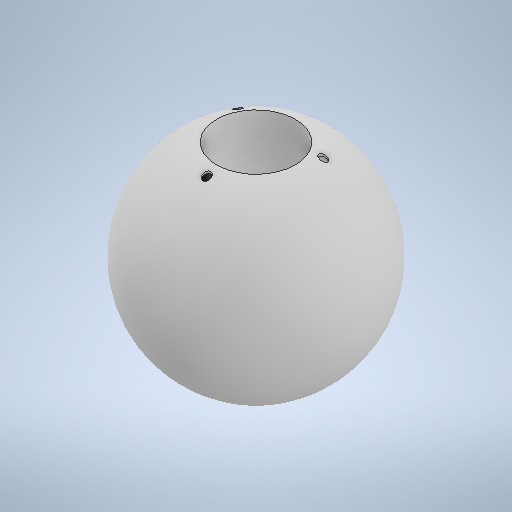
# Autodesk Inventor part: Buoy 10 2in Sphere
Saved by Autodesk Inventor 2025 (Build 290162000, 162)
## iProperties
Created: 2024-07-08
Part Number: Buoy 10 2in Sphere
Material: Generic
Document SubType Name: Modeling
Designer: track
Density: 1 g/cm^3
Appearance: Default
Mass: 1796.3 g
Surface Area: 1146.89 cm^2
Volume: 1796.3 cm^3
Author: track
## iProperties of the stored document Buoy 10 2in Sphere_3DPrint.ipt
Created: 2024-07-08
Part Number: Buoy 10 2in Sphere_3DPrint
Material: Generic
Document SubType Name: Modeling
Designer: track
Density: 1 g/cm^3
Appearance: Default
Author: track
Autodesk Inventor part; units mm, degrees
ref_plane "YZ Plane" through (0, 0, 0) normal (1, 0, 0) x (0, 1, 0)
ref_plane "XZ Plane" through (0, 0, 0) normal (0, 1, 0) x (-1, 0, 0)
ref_plane "XY Plane" through (0, 0, 0) normal (0, 0, 1) x (1, 0, 0)
sketch "Sketch1" plane through (0, 0, 0) normal (0, 0, 1) x (1, 0, 0)
  line L0 (0, 0) -> (0, 152.4)
  line L1 (0, 152.4) -> (30.48, 152.4) construction
  line L2 (30.48, 152.4) -> (30.48, 0)
  arc A0 (30.48, 0) -> (30.48, 152.4) centre (-1.27, 76.2) ccw
  line L3 (31.98, 2.2842) -> (31.98, 150.1158)
  arc A1 (31.98, 2.2842) -> (31.98, 150.1158) centre (-1.27, 76.2) ccw
  point P0 (81.28, 76.2)
  dimension "d0" = 152.4
  dimension "d1" = 30.48
  dimension "d2" = 50.8
  dimension "d3" = 0
  dimension "d4" = 1.5
  constraints: 8 end point, 5 point on circle, 2 centre point, 2 perpendicular, 1 vertical, 1 other
  measures "d0" distance of L1.end L2.end
  measures "d1" distance between parallel lines of L2 L0
  measures "d2" distance from line of L2 point (81.28, 76.2)
  measures "d3" vertical distance of L0.start L2.end
  measures "d4" distance between parallel lines of L2 L3
revolve "Revolution1" add sketch "Sketch1" angle 360 about axis through (0, 0, 0) along (0, 1, 0)
sketch "Sketch2" plane through (0, 0, 0) normal (0, 1, 0) x (-1, 0, 0)
  line L0 (0, 0) -> (0, 38.1) construction
  circle A0 centre (0, 38.1) radius 3
  dimension "d6" = 6
  dimension "d7" = 38.1
  constraints: 2 end point, 1 centre point, 1 coincident, 1 vertical
  measures "d6" diameter of A0
  measures "d7" distance of L0.start L0.end
extrude "Extrusion1" cut sketch "Sketch2" along normal through all
pattern_circular "Circular Pattern1" count 3 over 360 about axis through (0, 76.2, 0) along (0, 1, 0) of "Extrusion1"
body "Solid1"
